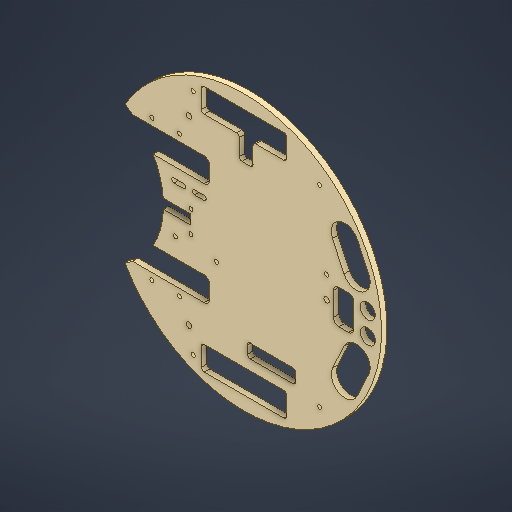
# Autodesk Inventor part: middle panel
Saved by Autodesk Inventor 2026.1 (Build 301233000, 233)
## iProperties
Created: 2025-03-16
Part Number: middle panel
Material: Generisch
Document SubType Name: Modeling
Designer: sfz
Density: 1 g/cm^3
Appearance: Beige
Author: sfz
Autodesk Inventor part; units mm, degrees
ref_plane "YZ Plane" through (0, 0, 0) normal (1, 0, 0) x (0, 1, 0)
ref_plane "XZ Plane" through (0, 0, 0) normal (0, 1, 0) x (-1, 0, 0)
ref_plane "XY Plane" through (0, 0, 0) normal (0, 0, 1) x (1, 0, 0)
sketch "Skizze1" plane through (0, 0, 0) normal (0, 1, 0) x (-1, 0, 0)
  arc A0 (86.6025, 50) -> (86.6025, -50) centre (117.2454, 0) ccw
  arc A1 (86.6025, 50) -> (86.6025, -50) centre (0, 0) ccw
  line L0 (31, -90) -> (-31, -90)
  line L1 (-31, -90) -> (-31, -72.5)
  line L2 (-31, -72.5) -> (31, -72.5)
  line L3 (31, -72.5) -> (31, -90)
  line L4 (31, 72.5) -> (-31, 72.5)
  line L5 (-31, 72.5) -> (-31, 90)
  line L6 (-31, 90) -> (31, 90)
  line L7 (31, 90) -> (31, 72.5)
  circle A2 centre (67, -51.25) radius 1.5
  circle A3 centre (47, -51.25) radius 1.5
  circle A4 centre (67, 51.25) radius 1.5
  circle A5 centre (47, 51.25) radius 1.5
  line L8 (81.191, -46.25) -> (25, -46.25)
  line L9 (25, -46.25) -> (25, -28.75)
  line L10 (25, -28.75) -> (66.1335, -28.75)
  line L11 (66.1335, 28.75) -> (25, 28.75)
  line L12 (25, 28.75) -> (25, 46.25)
  line L13 (25, 46.25) -> (81.191, 46.25)
  circle A6 centre (38.6025, -8) radius 1.5
  circle A7 centre (38.6025, 8) radius 1.5
  line L14 (58.7952, 4.75) -> (38.6457, 4.75)
  line L15 (38.6457, 4.75) -> (38.6457, -2.25)
  line L16 (38.6457, -2.25) -> (58.6457, -2.25)
  line L17 (-80, -12.5) -> (-65, -12.5)
  line L18 (-65, -12.5) -> (-65, 12.5)
  line L19 (-65, 12.5) -> (-80, 12.5)
  line L20 (-80, 12.5) -> (-80, -12.5)
  circle A8 centre (50, -15) radius 1.5
  circle A9 centre (-55, -70) radius 1.5
  circle A10 centre (-55, 70) radius 1.5
  circle A11 centre (37, -83) radius 1.5
  circle A12 centre (37, 83) radius 1.5
  line L21 (-73.4, -45.0752) -> (-81.8, -26.9248) construction
  line L22 (-64.3248, -40.8752) -> (-72.7248, -22.7248)
  line L23 (-90.8752, -31.1248) -> (-82.4752, -49.2752)
  arc A13 (-82.4752, -49.2752) -> (-64.3248, -40.8752) centre (-73.4, -45.0752) ccw
  arc A14 (-72.7248, -22.7248) -> (-90.8752, -31.1248) centre (-81.8, -26.9248) ccw
  line L24 (-73.4, -45.0752) -> (-81.8, -26.9248) construction
  line L25 (-81.8, 26.9248) -> (-73.4, 45.0752) construction
  line L26 (-90.8752, 31.1248) -> (-82.4752, 49.2752)
  line L27 (-64.3248, 40.8752) -> (-72.7248, 22.7248)
  arc A15 (-90.8752, 31.1248) -> (-72.7248, 22.7248) centre (-81.8, 26.9248) ccw
  arc A16 (-64.3248, 40.8752) -> (-82.4752, 49.2752) centre (-73.4, 45.0752) ccw
  line L28 (-81.8, 26.9248) -> (-73.4, 45.0752) construction
  circle A17 centre (20, -16) radius 1.5
  circle A18 centre (-60, 16) radius 1.5
  line L29 (-2.5, -65) -> (-37.5, -65)
  line L30 (-37.5, -65) -> (-37.5, -55)
  line L31 (-37.5, -55) -> (-2.5, -55)
  line L32 (-2.5, -55) -> (-2.5, -65)
  circle A19 centre (-90, -8) radius 5.5
  circle A20 centre (-90, 8) radius 5.5
  line L33 (3.5, 72.5) -> (-6.5, 72.5)
  line L34 (-6.5, 72.5) -> (-6.5, 56.5)
  line L35 (-6.5, 56.5) -> (3.5, 56.5)
  line L36 (3.5, 56.5) -> (3.5, 72.5)
  line L37 (36, 19.75) -> (29, 19.75) construction
  line L38 (36, 21.35) -> (29, 21.35)
  line L39 (29, 18.15) -> (36, 18.15)
  arc A21 (36, 18.15) -> (36, 21.35) centre (36, 19.75) ccw
  arc A22 (29, 21.35) -> (29, 18.15) centre (29, 19.75) ccw
  line L40 (44, 19.75) -> (51, 19.75) construction
  line L41 (44, 21.35) -> (51, 21.35)
  line L42 (51, 18.15) -> (44, 18.15)
  arc A23 (44, 21.35) -> (44, 18.15) centre (44, 19.75) ccw
  arc A24 (51, 18.15) -> (51, 21.35) centre (51, 19.75) ccw
  circle A25 centre (40, -66) radius 2
  circle A26 centre (40, 66) radius 2
  circle A27 centre (-60, 0) radius 2
  point P0 (58.6025, 0)
  point P1 (-31, -81.25)
  point P2 (-31, 81.25)
  point P3 (-77.6, -36)
  point P4 (-77.6, -36)
  point P5 (-77.6, 36)
  point P6 (-77.6, 36)
  point P7 (32.5, 19.75)
  point P8 (47.5, 19.75)
  dimension "d1" = 100
  dimension "d3" = 28
  dimension "d11" = 17.5
  dimension "d12" = 17.5
  dimension "d13" = 72.5
  dimension "d14" = 72.5
  dimension "d15" = 62
  dimension "d16" = 62
  dimension "d17" = 31
  dimension "d18" = 3
  dimension "d19" = 3
  dimension "d20" = 3
  dimension "d21" = 3
  dimension "d22" = 20
  dimension "d23" = 20
  dimension "d25" = 17.5
  dimension "d26" = 17.5
  dimension "d27" = 46.25
  dimension "d28" = 46.25
  dimension "d31" = 5
  dimension "d32" = 5
  dimension "d33" = 25
  dimension "d34" = 47
  dimension "d35" = 3
  dimension "d36" = 3
  dimension "d37" = 16
  dimension "d38" = 8
  dimension "d39" = 20
  dimension "d50" = 7
  dimension "d51" = 47.75
  dimension "d52" = 20
  dimension "d53" = 15
  dimension "d54" = 25
  dimension "d55" = 12.5
  dimension "d57" = 65
  dimension "d100" = 3
  dimension "d101" = 3
  dimension "d102" = 3
  dimension "d103" = 3
  dimension "d104" = 3
  dimension "d105" = 70
  dimension "d106" = 70
  dimension "d107" = 55
  dimension "d108" = 83
  dimension "d109" = 83
  dimension "d110" = 37
  dimension "d111" = 50
  dimension "d112" = 15
  dimension "d113" = 20
  dimension "d114" = 20
  dimension "d115" = 10
  dimension "d117" = 10
  dimension "d119" = 77.6
  dimension "d120" = 73.4
  dimension "d121" = 36
  dimension "d122" = 36
  dimension "d125" = 16
  dimension "d126" = 20
  dimension "d127" = 3
  dimension "d128" = 3
  dimension "d129" = 80
  dimension "d130" = 32
  dimension "d132" = 10
  dimension "d133" = 35
  constraints: 98 end point, 27 centre point, 18 point on circle, 17 equal length, 16 tangent, 10 perpendicular, 9 vertical alignment, 8 horizontal, 8 midpoint, 6 horizontal alignment, 5 point on line, 3 coincident, 11 other
  measures "d1" distance of A1.start A1.end
  measures "d3" horizontal distance of point (58.603, 0) A1.end
  measures "d11" distance of L6.end L4.start
  measures "d12" distance of L2.end L0.start
  measures "d13" distance from line of L2 A1.centre
  measures "d14" distance from line of A1.centre L4
  measures "d15" distance between parallel lines of L5 L7
  measures "d16" distance between parallel lines of L1 L3
  measures "d17" distance from line of L1 A1.centre
  measures "d18" diameter of A4
  measures "d19" diameter of A5
  measures "d20" diameter of A2
  measures "d21" diameter of A3
  measures "d22" distance of A3.centre A2.centre
  measures "d23" distance of A5.centre A4.centre
  measures "d25" distance between parallel lines of L11 L13
  measures "d26" distance between parallel lines of L8 L10
  measures "d27" distance from line of L8 A1.centre
  measures "d28" distance from line of A1.centre L13
  measures "d31" distance from line of L13 A5.centre
  measures "d32" distance from line of L8 A3.centre
  measures "d33" distance from line of point (0, 0) L12
  measures "d34" horizontal distance of point (0, 0) A5.centre
  measures "d35" diameter of A6
  measures "d36" diameter of A7
  measures "d37" distance of A6.centre A7.centre
  measures "d38" vertical distance of A1.centre A7.centre
  measures "d39" horizontal distance of point (58.603, 0) A7.centre
  measures "d50" distance of L14.end L15.end
  measures "d51" vertical distance of A1.end L16.end
  measures "d52" distance of L15.end L16.end
  measures "d53" distance of L18.end L19.end
  measures "d54" distance of L17.end L18.end
  measures "d55" distance from line of L19 A1.centre
  measures "d57" distance from line of point (0, 0) L18
  measures "d100" diameter of A11
  measures "d101" diameter of A9
  measures "d102" diameter of A10
  measures "d103" diameter of A12
  measures "d104" diameter of A8
  measures "d105" vertical distance of A1.centre A9.centre
  measures "d106" vertical distance of A10.centre A1.centre
  measures "d107" horizontal distance of A1.centre A10.centre
  measures "d108" vertical distance of A1.centre A12.centre
  measures "d109" vertical distance of A1.centre A11.centre
  measures "d110" horizontal distance of A1.centre A11.centre
  measures "d111" horizontal distance of A1.centre A8.centre
  measures "d112" vertical distance of point (58.603, 0) A8.centre
  measures "d113" distance of L21.end L21.start
  measures "d114" distance of L25.start L25.end
  measures "d115" radius of A16
  measures "d117" radius of A14
  measures "d119" horizontal distance of point (0, 0) point (-77.6, 36)
  measures "d120" horizontal distance of L25.end A1.centre
  measures "d121" vertical distance of point (-77.6, 36) A1.centre
  measures "d122" vertical distance of point (-77.6, -36) A1.centre
  measures "d125" vertical distance of point (0, 0) A17.centre
  measures "d126" horizontal distance of point (0, 0) A17.centre
  measures "d127" diameter of A17
  measures "d128" diameter of A18
  measures "d129" horizontal distance of A18.centre A17.centre
  measures "d130" vertical distance of A17.centre A18.centre
  measures "d132" distance of L31.end L29.start
  measures "d133" distance of L30.end L31.end
extrude "Extrusion1" add sketch "Skizze1" along normal blind 4 contours A0 L13 L12 L11 L14 L15 L16 L10 L9 L8 A1
fillet "Rundung1" radius 4 8 edges at (65, 2, 12.5) (65, 2, -12.5) (80, 2, 12.5) (80, 2, -12.5) (-25, 2, -28.75) (-25, 2, -46.25) (-25, 2, 28.75) (-25, 2, 46.25)
fillet "Rundung2" radius 2 16 edges at (31, 2, 90) (31, 2, 72.5) (-31, 2, 72.5) (-31, 2, 90) (31, 2, -90) (31, 2, -72.5) (-31, 2, -90) (-31, 2, -72.5) (2.5, 2, -55) (37.5, 2, -55) (37.5, 2, -65) (2.5, 2, -65) (6.5, 2, 56.5) (-3.5, 2, 56.5) (-3.5, 2, 72.5) (6.5, 2, 72.5)
equation "\"d14\" = d13"
equation "\"d15\" = d16"
